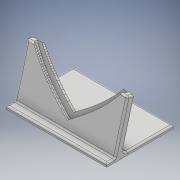
# Autodesk Inventor part: Supporto5
Saved by Autodesk Inventor 2018 (Build 220112000, 112)
## iProperties
Created: 2020-01-19
Part Number: Supporto5
Material: Generic
Document SubType Name: Modeling
Designer: Lorenzo Spadaro
Density: 1 g/cm^3
Appearance: Default
Author: Lorenzo Spadaro
Autodesk Inventor part; units mm, degrees
ref_plane "YZ Plane" through (0, 0, 0) normal (1, 0, 0) x (0, 1, 0)
ref_plane "XZ Plane" through (0, 0, 0) normal (0, 1, 0) x (-1, 0, 0)
ref_plane "XY Plane" through (0, 0, 0) normal (0, 0, 1) x (1, 0, 0)
sketch "Sketch1" plane through (0, 0, 0) normal (0, 0, 1) x (1, 0, 0)
  line L0 (-30, -20) -> (30, -20)
  line L1 (30, -20) -> (30, 20)
  line L2 (30, 20) -> (-30, 20)
  line L3 (-30, 20) -> (-30, -20)
  line L4 (-30, -20) -> (30, 20) construction
  line L5 (30, -20) -> (-30, 20) construction
  point P0 (0, 0)
  dimension "d0" = 60
  dimension "d1" = 40
  constraints: 12 end point, 2 midpoint, 2 parallel, 1 horizontal, 1 perpendicular
  measures "d0" distance of L2.end L1.end
  measures "d1" distance of L1.end L0.end
extrude "Extrusion1" add sketch "Sketch1" along normal blind 3
sketch "Sketch2" plane through (-30, -20, 0) normal (-1, 0, 0) x (0, 0, 1)
  line L0 (0, 0) -> (0, 40)
  line L1 (3, 40) -> (0, 40)
  line L2 (0, 40) -> (0, 0)
  line L3 (0, 0) -> (3, 0)
  line L4 (0, 40) -> (0, 20)
  line L5 (3, 40) -> (3, 5)
  line L6 (3, 5) -> (0, 5)
  line L7 (3, 0) -> (3, 40)
  line L8 (3, 5) -> (3, 0)
  line L9 (3, 5) -> (3, 9.805)
  line L10 (3, 9.805) -> (6, 9.805) construction
  line L11 (6.282765, 5.879614) -> (3, 5)
  line L12 (6.282765, 5.879614) -> (5.230961, 9.805)
  line L13 (6.282765, 5.879614) -> (10.346623, 5.879614) construction
  line L14 (5.230961, 9.805) -> (3, 9.805)
  dimension "d5" = 35
  dimension "d19" = 105
  dimension "d26" = 4.805
  dimension "d27" = 105
  constraints: 26 end point, 3 collinear, 3 horizontal, 3 point on line, 2 perpendicular, 1 equal length, 1 vertical
  measures "d5" distance of L1.start L5.end
  measures "d19" angle of L13 L12
  measures "d26" distance from line of L5.end L10
  measures "d27" angle of L7 L11
extrude "Extrusion2" add sketch "Sketch2" against normal blind 60 contours L5 L14 L12 L11
sketch "Sketch3" plane through (-30, -15, 3) normal (0, -0.9659258, 0.258819) x (1, 0, 0)
  line L0 (0, 3.398568) -> (60, 3.398568)
  line L1 (12.592311, 64.303412) -> (12.958694, 64.332521)
  line L2 (12.958694, 64.332521) -> (15.177373, 64.415061)
  line L3 (15.177373, 64.415061) -> (16.661991, 64.365177)
  line L4 (16.661991, 64.365177) -> (17.769726, 64.261939)
  line L5 (17.769726, 64.261939) -> (18.867022, 64.095258)
  line L6 (18.867022, 64.095258) -> (19.590244, 63.945636)
  line L7 (19.590244, 63.945636) -> (20.305002, 63.763178)
  line L8 (20.305002, 63.763178) -> (21.009903, 63.54578)
  line L9 (21.009903, 63.54578) -> (21.703356, 63.291635)
  line L10 (21.703356, 63.291635) -> (22.383868, 62.998836)
  line L11 (22.383868, 62.998836) -> (23.049947, 62.665577)
  line L12 (23.049947, 62.665577) -> (23.331467, 62.515535)
  line L13 (23.331467, 62.515535) -> (24.149779, 62.028902)
  line L14 (24.149779, 62.028902) -> (25.185077, 61.30316)
  line L15 (25.185077, 61.30316) -> (26.400848, 60.29306)
  line L16 (26.400848, 60.29306) -> (29.885544, 56.611384)
  line L17 (29.885544, 56.611384) -> (33.703552, 60.647146)
  line L18 (33.703552, 60.647146) -> (35.076276, 61.73641)
  line L19 (35.076276, 61.73641) -> (36.056629, 62.380953)
  line L20 (36.056629, 62.380953) -> (36.398998, 62.583466)
  line L21 (36.398998, 62.583466) -> (36.746215, 62.774297)
  line L22 (36.746215, 62.774297) -> (37.098078, 62.953848)
  line L23 (37.098078, 62.953848) -> (37.454288, 63.122217)
  line L24 (37.454288, 63.122217) -> (37.814542, 63.279703)
  line L25 (37.814542, 63.279703) -> (38.54658, 63.563221)
  line L26 (38.54658, 63.563221) -> (39.292386, 63.806195)
  line L27 (39.292386, 63.806195) -> (40.050049, 64.010818)
  line L28 (40.050049, 64.010818) -> (40.817863, 64.178882)
  line L29 (40.817863, 64.178882) -> (41.59382, 64.31238)
  line L30 (41.59382, 64.31238) -> (42.376111, 64.413403)
  line L31 (42.376111, 64.413403) -> (43.55743, 64.50827)
  line L32 (43.55743, 64.50827) -> (45.137415, 64.539379)
  line L33 (45.137415, 64.539379) -> (47.099711, 64.447361)
  line L34 (47.099711, 64.447361) -> (47.482254, 64.413437)
  line L35 (47.482254, 64.413437) -> (47.862944, 64.368005)
  line L36 (47.862944, 64.368005) -> (48.24148, 64.311464)
  line L37 (48.24148, 64.311464) -> (48.991688, 64.165553)
  line L38 (48.991688, 64.165553) -> (49.73137, 63.977198)
  line L39 (49.73137, 63.977198) -> (50.45922, 63.748095)
  line L40 (50.45922, 63.748095) -> (51.173731, 63.479836)
  line L41 (51.173731, 63.479836) -> (51.873497, 63.174016)
  line L42 (51.873497, 63.174016) -> (52.55711, 62.832229)
  line L43 (52.55711, 62.832229) -> (53.223066, 62.456069)
  line L44 (53.223066, 62.456069) -> (53.870055, 62.047231)
  line L45 (53.870055, 62.047231) -> (54.496573, 61.607208)
  line L46 (54.496573, 61.607208) -> (55.101212, 61.137695)
  line L47 (55.101212, 61.137695) -> (55.682567, 60.640185)
  line L48 (55.682567, 60.640185) -> (56.239229, 60.116474)
  line L49 (56.239229, 60.116474) -> (56.769693, 59.567954)
  line L50 (56.769693, 59.567954) -> (57.086721, 59.221957)
  line L51 (57.086721, 59.221957) -> (57.393082, 58.867816)
  line L52 (57.393082, 58.867816) -> (57.688776, 58.505831)
  line L53 (57.688776, 58.505831) -> (57.973892, 58.136396)
  line L54 (57.973892, 58.136396) -> (58.248465, 57.759638)
  line L55 (58.248465, 57.759638) -> (58.512767, 57.376037)
  line L56 (58.512767, 57.376037) -> (58.766597, 56.985692)
  line L57 (58.766597, 56.985692) -> (59.010253, 56.589105)
  line L58 (59.010253, 56.589105) -> (59.243835, 56.186375)
  line L59 (59.243835, 56.186375) -> (59.46724, 55.777903)
  line L60 (59.46724, 55.777903) -> (59.680669, 55.36389)
  line L61 (59.680669, 55.36389) -> (60.077988, 54.520739)
  line L62 (60.077988, 54.520739) -> (60.436185, 53.659126)
  line L63 (60.436185, 53.659126) -> (60.756147, 52.781552)
  line L64 (60.756147, 52.781552) -> (61.038466, 51.890322)
  line L65 (61.038466, 51.890322) -> (61.283833, 50.987737)
  line L66 (61.283833, 50.987737) -> (61.492836, 50.076101)
  line L67 (61.492836, 50.076101) -> (61.666167, 49.157916)
  line L68 (61.666167, 49.157916) -> (61.804515, 48.235385)
  line L69 (61.804515, 48.235385) -> (61.908472, 47.31091)
  line L70 (61.908472, 47.31091) -> (61.925428, 43.259027)
  line L71 (61.925428, 43.259027) -> (61.867686, 42.674287)
  line L72 (61.867686, 42.674287) -> (61.795735, 42.088881)
  line L73 (61.795735, 42.088881) -> (61.710172, 41.506318)
  line L74 (61.710172, 41.506318) -> (61.611397, 40.9266)
  line L75 (61.611397, 40.9266) -> (61.49971, 40.349827)
  line L76 (61.49971, 40.349827) -> (61.37541, 39.776102)
  line L77 (61.37541, 39.776102) -> (61.238797, 39.205425)
  line L78 (61.238797, 39.205425) -> (61.09027, 38.637999)
  line L79 (61.09027, 38.637999) -> (60.92993, 38.073723)
  line L80 (60.92993, 38.073723) -> (60.758376, 37.5127)
  line L81 (60.758376, 37.5127) -> (60.575708, 36.955031)
  line L82 (60.575708, 36.955031) -> (60.178429, 35.850058)
  line L83 (60.178429, 35.850058) -> (59.740789, 34.759417)
  line L84 (59.740789, 34.759417) -> (59.265187, 33.683618)
  line L85 (59.265187, 33.683618) -> (58.754121, 32.62307)
  line L86 (58.754121, 32.62307) -> (58.210087, 31.578484)
  line L87 (58.210087, 31.578484) -> (57.635685, 30.550371)
  line L88 (57.635685, 30.550371) -> (56.722496, 29.040236)
  line L89 (56.722496, 29.040236) -> (55.754839, 27.570274)
  line L90 (55.754839, 27.570274) -> (55.262169, 26.869206)
  line L91 (55.262169, 26.869206) -> (54.759665, 26.176097)
  line L92 (54.759665, 26.176097) -> (54.247729, 25.490649)
  line L93 (54.247729, 25.490649) -> (53.726461, 24.812762)
  line L94 (53.726461, 24.812762) -> (53.196262, 24.142237)
  line L95 (53.196262, 24.142237) -> (52.110275, 22.822781)
  line L96 (52.110275, 22.822781) -> (50.991771, 21.530989)
  line L97 (50.991771, 21.530989) -> (49.843056, 20.265571)
  line L98 (49.843056, 20.265571) -> (48.666436, 19.025336)
  line L99 (48.666436, 19.025336) -> (47.464115, 17.808994)
  line L100 (47.464115, 17.808994) -> (45.617358, 16.02655)
  line L101 (45.617358, 16.02655) -> (43.725406, 14.290617)
  line L102 (43.725406, 14.290617) -> (40.492299, 11.489663)
  line L103 (40.492299, 11.489663) -> (38.516713, 9.857281)
  line L104 (38.516713, 9.857281) -> (30.108542, 3.524339)
  line L105 (30.108542, 3.524339) -> (25.613236, 6.766256)
  line L106 (25.613236, 6.766256) -> (22.956408, 8.774555)
  line L107 (22.956408, 8.774555) -> (21.20846, 10.144353)
  line L108 (21.20846, 10.144353) -> (19.4827, 11.541243)
  line L109 (19.4827, 11.541243) -> (17.782216, 12.967639)
  line L110 (17.782216, 12.967639) -> (16.1101, 14.425454)
  line L111 (16.1101, 14.425454) -> (15.28559, 15.166911)
  line L112 (15.28559, 15.166911) -> (14.469444, 15.917102)
  line L113 (14.469444, 15.917102) -> (13.66186, 16.676229)
  line L114 (13.66186, 16.676229) -> (12.863337, 17.444594)
  line L115 (12.863337, 17.444594) -> (12.074175, 18.222498)
  line L116 (12.074175, 18.222498) -> (11.294772, 19.010244)
  line L117 (11.294772, 19.010244) -> (10.525626, 19.808032)
  line L118 (10.525626, 19.808032) -> (9.767038, 20.616064)
  line L119 (9.767038, 20.616064) -> (9.019406, 21.434743)
  line L120 (9.019406, 21.434743) -> (8.283128, 22.264369)
  line L121 (8.283128, 22.264369) -> (7.558503, 23.105044)
  line L122 (7.558503, 23.105044) -> (6.846031, 23.95717)
  line L123 (6.846031, 23.95717) -> (6.14611, 24.821048)
  line L124 (6.14611, 24.821048) -> (5.295269, 25.928197)
  line L125 (5.295269, 25.928197) -> (4.470723, 27.060657)
  line L126 (4.470723, 27.060657) -> (3.676074, 28.217642)
  line L127 (3.676074, 28.217642) -> (2.915326, 29.398568)
  line L128 (2.915326, 29.398568) -> (2.548714, 29.997939)
  line L129 (2.548714, 29.997939) -> (2.192079, 30.603052)
  line L130 (2.192079, 30.603052) -> (1.845719, 31.213908)
  line L131 (1.845719, 31.213908) -> (1.510336, 31.83041)
  line L132 (1.510336, 31.83041) -> (1.186131, 32.452459)
  line L133 (1.186131, 32.452459) -> (0.873701, 33.080057)
  line L134 (0.873701, 33.080057) -> (0.57365, 33.713107)
  line L135 (0.57365, 33.713107) -> (0.286176, 34.351509)
  line L136 (0.286176, 34.351509) -> (0.01208, 34.995168)
  line L137 (0.01208, 34.995168) -> (-0.248439, 35.644183)
  line L138 (-0.248439, 35.644183) -> (-0.494778, 36.298258)
  line L139 (-0.494778, 36.298258) -> (-0.726439, 36.957495)
  line L140 (-0.726439, 36.957495) -> (-0.94302, 37.621694)
  line L141 (-0.94302, 37.621694) -> (-1.144022, 38.290859)
  line L142 (-1.144022, 38.290859) -> (-1.328845, 38.964891)
  line L143 (-1.328845, 38.964891) -> (-1.497187, 39.643693)
  line L144 (-1.497187, 39.643693) -> (-1.648549, 40.327365)
  line L145 (-1.648549, 40.327365) -> (-1.78243, 41.015611)
  line L146 (-1.78243, 41.015611) -> (-1.898231, 41.708532)
  line L147 (-1.898231, 41.708532) -> (-1.99565, 42.405931)
  line L148 (-1.99565, 42.405931) -> (-2.074088, 43.107809)
  line L149 (-2.074088, 43.107809) -> (-2.089544, 46.801076)
  line L150 (-2.089544, 46.801076) -> (-1.961684, 48.029622)
  line L151 (-1.961684, 48.029622) -> (-1.776004, 49.25341)
  line L152 (-1.776004, 49.25341) -> (-1.530382, 50.467349)
  line L153 (-1.530382, 50.467349) -> (-1.222497, 51.666447)
  line L154 (-1.222497, 51.666447) -> (-0.85023, 52.846016)
  line L155 (-0.85023, 52.846016) -> (-0.565162, 53.619015)
  line L156 (-0.565162, 53.619015) -> (-0.249943, 54.379641)
  line L157 (-0.249943, 54.379641) -> (0.096236, 55.126296)
  line L158 (0.096236, 55.126296) -> (0.473978, 55.857784)
  line L159 (0.473978, 55.857784) -> (0.883891, 56.572405)
  line L160 (0.883891, 56.572405) -> (1.326681, 57.268764)
  line L161 (1.326681, 57.268764) -> (1.802953, 57.945463)
  line L162 (1.802953, 57.945463) -> (2.070477, 58.298886)
  line L163 (2.070477, 58.298886) -> (2.347528, 58.645648)
  line L164 (2.347528, 58.645648) -> (2.634008, 58.98545)
  line L165 (2.634008, 58.98545) -> (2.929719, 59.317991)
  line L166 (2.929719, 59.317991) -> (3.234362, 59.642968)
  line L167 (3.234362, 59.642968) -> (3.547638, 59.960082)
  line L168 (3.547638, 59.960082) -> (3.869349, 60.268831)
  line L169 (3.869349, 60.268831) -> (4.199195, 60.569114)
  line L170 (4.199195, 60.569114) -> (4.537079, 60.860431)
  line L171 (4.537079, 60.860431) -> (4.882701, 61.142479)
  line L172 (4.882701, 61.142479) -> (5.235764, 61.414959)
  line L173 (5.235764, 61.414959) -> (5.595969, 61.677469)
  line L174 (5.595969, 61.677469) -> (5.963333, 61.929784)
  line L175 (5.963333, 61.929784) -> (6.33734, 62.171527)
  line L176 (6.33734, 62.171527) -> (6.717792, 62.402396)
  line L177 (6.717792, 62.402396) -> (7.104591, 62.621991)
  line L178 (7.104591, 62.621991) -> (7.497437, 62.830012)
  line L179 (7.497437, 62.830012) -> (7.896033, 63.026155)
  line L180 (7.896033, 63.026155) -> (8.300079, 63.210021)
  line L181 (8.300079, 63.210021) -> (8.709476, 63.381409)
  line L182 (8.709476, 63.381409) -> (9.123927, 63.539818)
  line L183 (9.123927, 63.539818) -> (9.543232, 63.685046)
  line L184 (9.543232, 63.685046) -> (9.966994, 63.816693)
  line L185 (9.966994, 63.816693) -> (10.395212, 63.934458)
  line L186 (10.395212, 63.934458) -> (10.827389, 64.038039)
  line L187 (10.827389, 64.038039) -> (11.263526, 64.127036)
  line L188 (11.263526, 64.127036) -> (11.703125, 64.201148)
  line L189 (11.703125, 64.201148) -> (12.146186, 64.260074)
  line L190 (12.146186, 64.260074) -> (12.592311, 64.303412)
  line L191 (0, 0) -> (0, 3.398568)
  line L192 (0, 3.398568) -> (0, 29.398568)
  line L193 (0, 29.398568) -> (2.915326, 29.398568)
  line L194 (60, 3.398568) -> (60, 0)
  line L195 (60, 3.398568) -> (60, 29.398568)
  line L196 (60, 29.398568) -> (56.939182, 29.398568)
  point P0 (30, 0.984508)
  dimension "d15" = 26
  dimension "d16" = 26
  constraints: 388 end point, 4 perpendicular, 2 point on line, 1 horizontal, 1 parallel, 1 vertical
  measures "d15" distance of L0.start L192.end
  measures "d16" distance of L0.end L195.end
extrude "Extrusion3" add sketch "Sketch3" against normal blind 3.1 contours L192 L193 L127 L126 L125 L124 L123 L122 L121 L120 L119 L118 L117 L116 L115 L114 L113 L112 L111 L110 L109 L108 L107 L106 L105 L104 L103 L102 L101 L100 L99 L98 L97 L96 L95 L94 L93 L92 L91 L90 L89 L88 L196 L195 L0
sketch "Sketch4" plane through (26.939182, -7.391091, 31.396836) normal (0, 0.258819, 0.9659258) x (1, 0, 0)
  line L0 (3.060818, 3.1) -> (3.060818, 3.1)
  line L1 (-56.939182, 3.1) -> (-56.939182, 3.1)
  line L2 (-56.939182, 3.1) -> (3.060818, 3.1)
  line L3 (-56.939182, 5.40781) -> (3.060818, 5.40781)
  line L4 (-56.939182, 3.1) -> (-56.939182, 4.6)
  line L5 (-56.939182, 34.583861) -> (-56.939182, -4.053172)
  line L6 (-56.939182, 4.6) -> (3.060818, 4.6)
  line L7 (3.060818, 4.6) -> (3.060818, 3.1)
  line L8 (3.060818, -4.053172) -> (3.060818, 34.583861)
  point P0 (-26.939182, 15.265345)
  point P1 (-56.939182, 4.641274)
  point P2 (3.060818, 4.641274)
  dimension "d23" = 1.5
  constraints: 8 end point, 1 collinear, 1 perpendicular, 1 point on line
  measures "d23" distance of L1.start L4.end
extrude "Extrusion5" add sketch "Sketch4" against normal blind 28 contours L4 L6 L7 L2
sketch "Sketch6" plane through (-27.084674, -4.396721, 30.594497) normal (0, -0.9659258, 0.258819) x (1, 0, 0)
  line L0 (0, 0) -> (0.760749, -1.180927)
  line L1 (0.760749, -1.180927) -> (1.555397, -2.337911)
  line L2 (1.555397, -2.337911) -> (2.379944, -3.470371)
  line L3 (0, 0) -> (0.760749, -1.180927)
  line L4 (0.760749, -1.180927) -> (1.555397, -2.337911)
  line L5 (1.555397, -2.337911) -> (2.379944, -3.470371)
  line L6 (2.379944, -3.470371) -> (3.230784, -4.57752)
  line L7 (3.230784, -4.57752) -> (3.930705, -5.441399)
  line L8 (3.930705, -5.441399) -> (4.643178, -6.293524)
  line L9 (4.643178, -6.293524) -> (5.367802, -7.134199)
  line L10 (5.367802, -7.134199) -> (6.10408, -7.963825)
  line L11 (6.10408, -7.963825) -> (6.851713, -8.782504)
  line L12 (6.851713, -8.782504) -> (7.610301, -9.590537)
  line L13 (7.610301, -9.590537) -> (8.379446, -10.388325)
  line L14 (8.379446, -10.388325) -> (9.15885, -11.17607)
  line L15 (9.15885, -11.17607) -> (9.948012, -11.953974)
  line L16 (9.948012, -11.953974) -> (10.746534, -12.72234)
  line L17 (10.746534, -12.72234) -> (11.554118, -13.481467)
  line L18 (11.554118, -13.481467) -> (12.370265, -14.231658)
  line L19 (12.370265, -14.231658) -> (13.194775, -14.973114)
  line L20 (13.194775, -14.973114) -> (14.86689, -16.430929)
  line L21 (14.86689, -16.430929) -> (16.567374, -17.857326)
  line L22 (16.567374, -17.857326) -> (18.293135, -19.254216)
  line L23 (18.293135, -19.254216) -> (20.041082, -20.624013)
  line L24 (20.041082, -20.624013) -> (22.69791, -22.632312)
  line L25 (22.69791, -22.632312) -> (27.193216, -25.874229)
  line L26 (27.193216, -25.874229) -> (35.601388, -19.541287)
  line L27 (35.601388, -19.541287) -> (37.576974, -17.908905)
  line L28 (37.576974, -17.908905) -> (40.810081, -15.107951)
  line L29 (40.810081, -15.107951) -> (42.702033, -13.372018)
  line L30 (42.702033, -13.372018) -> (44.54879, -11.589575)
  line L31 (44.54879, -11.589575) -> (45.75111, -10.373232)
  line L32 (45.75111, -10.373232) -> (46.927731, -9.132998)
  line L33 (46.927731, -9.132998) -> (48.076445, -7.867579)
  line L34 (48.076445, -7.867579) -> (49.194949, -6.575787)
  line L35 (49.194949, -6.575787) -> (50.280937, -5.256331)
  line L36 (50.280937, -5.256331) -> (50.811136, -4.585807)
  line L37 (50.811136, -4.585807) -> (51.332403, -3.907919)
  line L38 (51.332403, -3.907919) -> (51.844339, -3.222471)
  line L39 (51.844339, -3.222471) -> (52.346843, -2.529362)
  line L40 (52.346843, -2.529362) -> (52.839514, -1.828294)
  line L41 (52.839514, -1.828294) -> (53.807171, -0.358332)
  line L42 (53.807171, -0.358332) -> (54.023856, 0)
  line L43 (0, 0) -> (54.023856, 0)
  line L44 (0, 4) -> (0.760749, 2.819073)
  line L45 (0.760749, 2.819073) -> (1.555397, 1.662089)
  line L46 (1.555397, 1.662089) -> (2.379944, 0.529629)
  line L47 (0, 4) -> (0.760749, 2.819073)
  line L48 (0.760749, 2.819073) -> (1.555397, 1.662089)
  line L49 (1.555397, 1.662089) -> (2.379944, 0.529629)
  line L50 (2.379944, 0.529629) -> (3.230784, -0.57752)
  line L51 (3.230784, -0.57752) -> (3.930705, -1.441399)
  line L52 (3.930705, -1.441399) -> (4.643178, -2.293524)
  line L53 (4.643178, -2.293524) -> (5.367802, -3.134199)
  line L54 (5.367802, -3.134199) -> (6.10408, -3.963825)
  line L55 (6.10408, -3.963825) -> (6.851713, -4.782504)
  line L56 (6.851713, -4.782504) -> (7.610301, -5.590537)
  line L57 (7.610301, -5.590537) -> (8.379446, -6.388325)
  line L58 (8.379446, -6.388325) -> (9.15885, -7.17607)
  line L59 (9.15885, -7.17607) -> (9.948012, -7.953974)
  line L60 (9.948012, -7.953974) -> (10.746534, -8.72234)
  line L61 (10.746534, -8.72234) -> (11.554118, -9.481467)
  line L62 (11.554118, -9.481467) -> (12.370265, -10.231658)
  line L63 (12.370265, -10.231658) -> (13.194775, -10.973114)
  line L64 (13.194775, -10.973114) -> (14.86689, -12.430929)
  line L65 (14.86689, -12.430929) -> (16.567374, -13.857326)
  line L66 (16.567374, -13.857326) -> (18.293135, -15.254216)
  line L67 (18.293135, -15.254216) -> (20.041082, -16.624013)
  line L68 (20.041082, -16.624013) -> (22.69791, -18.632312)
  line L69 (22.69791, -18.632312) -> (27.193216, -21.874229)
  line L70 (27.193216, -21.874229) -> (35.601388, -15.541287)
  line L71 (35.601388, -15.541287) -> (37.576974, -13.908905)
  line L72 (37.576974, -13.908905) -> (40.810081, -11.107951)
  line L73 (40.810081, -11.107951) -> (42.702033, -9.372018)
  line L74 (42.702033, -9.372018) -> (44.54879, -7.589575)
  line L75 (44.54879, -7.589575) -> (45.75111, -6.373232)
  line L76 (45.75111, -6.373232) -> (46.927731, -5.132998)
  line L77 (46.927731, -5.132998) -> (48.076445, -3.867579)
  line L78 (48.076445, -3.867579) -> (49.194949, -2.575787)
  line L79 (49.194949, -2.575787) -> (50.280937, -1.256331)
  line L80 (50.280937, -1.256331) -> (50.811136, -0.585807)
  line L81 (50.811136, -0.585807) -> (51.332403, 0.092081)
  line L82 (51.332403, 0.092081) -> (51.844339, 0.777529)
  line L83 (51.844339, 0.777529) -> (52.346843, 1.470638)
  line L84 (52.346843, 1.470638) -> (52.839514, 2.171706)
  line L85 (52.839514, 2.171706) -> (53.807171, 3.641668)
  line L86 (27.193216, -21.874229) -> (27.193216, -25.874229)
  line L87 (0, 0) -> (54.023856, 0)
  line L88 (2.786962, 0) -> (51.261597, 0)
  point P0 (27.084674, -28.41406)
  dimension "d69" = 4
  constraints: 88 end point, 4 point on line
  measures "d69" distance of L25.end L70.start
extrude "Extrusion11" cut sketch "Sketch6" against normal up to next contours L43 L81 L80 L79 L78 L77 L76 L75 L74 L73 L72 L71 L70 L69 L68 L67 L66 L65 L64 L63 L62 L61 L60 L59 L58 L57 L56 L55 L54 L53 L52 L51 L50
sketch "Sketch11" plane through (-30, -15, 3) normal (0, -0.9659258, 0.258819) x (1, 0, 0)
  line L0 (3.676074, 28.217642) -> (2.915326, 29.398568)
  line L1 (4.470723, 27.060657) -> (3.676074, 28.217642)
  line L2 (5.295269, 25.928197) -> (4.470723, 27.060657)
  line L3 (6.14611, 24.821048) -> (5.295269, 25.928197)
  line L4 (6.846031, 23.95717) -> (6.14611, 24.821048)
  line L5 (7.558503, 23.105044) -> (6.846031, 23.95717)
  line L6 (8.283128, 22.264369) -> (7.558503, 23.105044)
  line L7 (9.019406, 21.434743) -> (8.283128, 22.264369)
  line L8 (9.767038, 20.616064) -> (9.019406, 21.434743)
  line L9 (10.525626, 19.808032) -> (9.767038, 20.616064)
  line L10 (11.294772, 19.010244) -> (10.525626, 19.808032)
  line L11 (12.074175, 18.222498) -> (11.294772, 19.010244)
  line L12 (12.863337, 17.444594) -> (12.074175, 18.222498)
  line L13 (14.469444, 15.917102) -> (13.66186, 16.676229)
  line L14 (13.66186, 16.676229) -> (12.863337, 17.444594)
  line L15 (15.28559, 15.166911) -> (14.469444, 15.917102)
  line L16 (16.1101, 14.425454) -> (15.28559, 15.166911)
  line L17 (17.782216, 12.967639) -> (16.1101, 14.425454)
  line L18 (19.4827, 11.541243) -> (17.782216, 12.967639)
  line L19 (21.20846, 10.144353) -> (19.4827, 11.541243)
  line L20 (22.956408, 8.774555) -> (21.20846, 10.144353)
  line L21 (25.613236, 6.766256) -> (22.956408, 8.774555)
  line L22 (30.108542, 3.524339) -> (25.613236, 6.766256)
  line L23 (38.516713, 9.857281) -> (30.108542, 3.524339)
  line L24 (40.492299, 11.489663) -> (38.516713, 9.857281)
  line L25 (43.725406, 14.290617) -> (40.492299, 11.489663)
  line L26 (45.617358, 16.02655) -> (43.725406, 14.290617)
  line L27 (47.464115, 17.808994) -> (45.617358, 16.02655)
  line L28 (48.666436, 19.025336) -> (47.464115, 17.808994)
  line L29 (49.843056, 20.265571) -> (48.666436, 19.025336)
  line L30 (50.991771, 21.530989) -> (49.843056, 20.265571)
  line L31 (52.110275, 22.822781) -> (50.991771, 21.530989)
  line L32 (53.196262, 24.142237) -> (52.110275, 22.822781)
  line L33 (53.726461, 24.812762) -> (53.196262, 24.142237)
  line L34 (54.247729, 25.490649) -> (53.726461, 24.812762)
  line L35 (54.759665, 26.176097) -> (54.247729, 25.490649)
  line L36 (55.262169, 26.869206) -> (54.759665, 26.176097)
  line L37 (55.754839, 27.570274) -> (55.262169, 26.869206)
  line L38 (56.722496, 29.040236) -> (55.754839, 27.570274)
  line L39 (56.939182, 29.398568) -> (56.722496, 29.040236)
  line L40 (25.613236, 6.766256) -> (30.108542, 3.524339)
  line L41 (30.108542, 3.524339) -> (30.108542, 4.524339)
  line L42 (30.108542, 3.524339) -> (31.108542, 3.524339) construction
  line L43 (3.676074, 29.217642) -> (2.915326, 30.398568)
  line L44 (4.470723, 28.060657) -> (3.676074, 29.217642)
  line L45 (5.295269, 26.928197) -> (4.470723, 28.060657)
  line L46 (6.14611, 25.821048) -> (5.295269, 26.928197)
  line L47 (6.846031, 24.95717) -> (6.14611, 25.821048)
  line L48 (7.558503, 24.105044) -> (6.846031, 24.95717)
  line L49 (8.283128, 23.264369) -> (7.558503, 24.105044)
  line L50 (9.019406, 22.434743) -> (8.283128, 23.264369)
  line L51 (9.767038, 21.616064) -> (9.019406, 22.434743)
  line L52 (10.525626, 20.808032) -> (9.767038, 21.616064)
  line L53 (11.294772, 20.010244) -> (10.525626, 20.808032)
  line L54 (12.074175, 19.222498) -> (11.294772, 20.010244)
  line L55 (12.863337, 18.444594) -> (12.074175, 19.222498)
  line L56 (14.469444, 16.917102) -> (13.66186, 17.676229)
  line L57 (13.66186, 17.676229) -> (12.863337, 18.444594)
  line L58 (15.28559, 16.166911) -> (14.469444, 16.917102)
  line L59 (16.1101, 15.425454) -> (15.28559, 16.166911)
  line L60 (17.782216, 13.967639) -> (16.1101, 15.425454)
  line L61 (19.4827, 12.541243) -> (17.782216, 13.967639)
  line L62 (21.20846, 11.144353) -> (19.4827, 12.541243)
  line L63 (22.956408, 9.774555) -> (21.20846, 11.144353)
  line L64 (25.613236, 7.766256) -> (22.956408, 9.774555)
  line L65 (30.108542, 4.524339) -> (25.613236, 7.766256)
  line L66 (38.516713, 10.857281) -> (30.108542, 4.524339)
  line L67 (40.492299, 12.489663) -> (38.516713, 10.857281)
  line L68 (43.725406, 15.290617) -> (40.492299, 12.489663)
  line L69 (45.617358, 17.02655) -> (43.725406, 15.290617)
  line L70 (47.464115, 18.808994) -> (45.617358, 17.02655)
  line L71 (48.666436, 20.025336) -> (47.464115, 18.808994)
  line L72 (49.843056, 21.265571) -> (48.666436, 20.025336)
  line L73 (50.991771, 22.530989) -> (49.843056, 21.265571)
  line L74 (52.110275, 23.822781) -> (50.991771, 22.530989)
  line L75 (53.196262, 25.142237) -> (52.110275, 23.822781)
  line L76 (53.726461, 25.812762) -> (53.196262, 25.142237)
  line L77 (54.247729, 26.490649) -> (53.726461, 25.812762)
  line L78 (54.759665, 27.176097) -> (54.247729, 26.490649)
  line L79 (55.262169, 27.869206) -> (54.759665, 27.176097)
  line L80 (55.754839, 28.570274) -> (55.262169, 27.869206)
  line L81 (56.722496, 30.040236) -> (55.754839, 28.570274)
  line L82 (56.939182, 30.398568) -> (56.722496, 30.040236)
  line L83 (2.915326, 29.398568) -> (3.559522, 29.398568)
  line L84 (56.939182, 29.398568) -> (56.300094, 29.398568)
  point P0 (30, 0.984508)
  dimension "d72" = 1
  dimension "d73" = 90
  constraints: 88 end point, 3 point on line, 2 horizontal, 1 perpendicular, 1 vertical
  measures "d72" distance of L22.start L41.end
  measures "d73" angle of L42 L41
extrude "Extrusion12" add sketch "Sketch11" against normal blind 1
sketch "Sketch8" plane through (0, 0, 3) normal (0, 0, 1) x (1, 0, 0)
  line L0 (24, -5.148917) -> (21, -5.148917)
  line L1 (21, -5.148917) -> (21, -7.148917)
  line L2 (21, -7.148917) -> (24, -7.148917)
  line L3 (24, -7.148917) -> (24, -5.148917)
  line L4 (-21, -5.148917) -> (-24, -5.148917)
  line L5 (-24, -5.148917) -> (-24, -7.147451)
  line L6 (-24, -7.147451) -> (-21, -7.147451)
  line L7 (-21, -7.147451) -> (-21, -5.148917)
  line L8 (-24, -5.148917) -> (-29, -5.148917)
  line L9 (29, -5.148917) -> (24, -5.148917)
  line L10 (29, -4.877374) -> (29, 20)
  line L11 (30, 20) -> (-30, 20)
  line L12 (-29, -5.148917) -> (-29, 20)
  line L13 (30, -10.195) -> (30, 20)
  line L14 (29, -4.877374) -> (29, -5.148917)
  line L15 (29, -5.148917) -> (29, -9.566685)
  line L16 (-29, -5.148917) -> (-29, -9.566685)
  line L17 (-29, -9.566685) -> (29, -9.566685)
  line L18 (29, -9.566685) -> (30, -9.566685)
  line L19 (-29, -9.566685) -> (-30, -9.566685)
  line L20 (-30, 20) -> (-30, -10.195)
  line L21 (-29, -9.566685) -> (-28, -9.566685) construction
  point P0 (0, 0)
  dimension "d51" = 3
  dimension "d52" = 2
  dimension "d53" = 3
  dimension "d54" = 42
  dimension "d55" = 3
  dimension "d56" = 5
  dimension "d62" = 27.14745
  dimension "d63" = 24.87737
  dimension "d76" = 180
  constraints: 38 end point, 9 perpendicular, 5 point on line, 3 vertical, 2 horizontal, 1 collinear, 1 parallel
  measures "d51" distance of L0.start L0.end
  measures "d52" distance of L0.end L1.end
  measures "d53" distance of L1.end L2.end
  measures "d54" distance of L0.end L4.start
  measures "d55" distance of L4.start L4.end
  measures "d56" distance of L4.end L8.end
  measures "d62" distance between parallel lines of L6 L11
  measures "d63" distance from line of L10.start L11
  measures "d76" angle of L19 L21
extrude "Extrusion9" add sketch "Sketch8" along normal up to next contours L3 L2 L1 L0 | L7 L6 L5 L4
sketch "Sketch10" plane through (0, 0, 0) normal (0, 0, -1) x (-1, 0, 0)
  line L0 (-30, 20) -> (30, 20)
  line L1 (-30, 20) -> (-30, -20)
  line L2 (-30, -20) -> (30, -20)
  line L3 (30, 20) -> (30, -20) projected
  line L4 (30, -20) -> (30, 20)
  point P0 (0, 0)
  constraints: 8 end point, 2 perpendicular, 1 vertical
extrude "Extrusion10" cut sketch "Sketch10" against normal blind 1
fillet "Fillet7" radius 0.5 16 edges at (-21, -5.1489, 12.4959) (-21, -7.1475, 8.7665) (-24, -5.1489, 12.4959) (-24, -7.1475, 8.7665) (21, -5.1489, 12.4959) (21, -7.1489, 8.7638) (24, -5.1489, 12.4959) (24, -7.1489, 8.7638) (24, -6.1489, 3) (22.5, -7.1489, 3) (21, -6.1489, 3) (22.5, -5.1489, 3) (-24, -6.1482, 3) (-22.5, -5.1489, 3) (-21, -6.1482, 3) (-22.5, -7.1475, 3)
fillet "Fillet9" radius 2 5 edges at (0, -10.195, 3) (0, -10.1948, 3.1603) (30, -10.1949, 3.1604) (-30, -10.1949, 3.1604) (0, -10.195, 3.1604)
fillet "Fillet10" radius 1 18 edges at (-30, 6.1844, 3) (-30, -6.2555, 17.862) (-30, -9.218, 3.7825) (0, 20, 3) (-30, -11.1955, 17.1984) (-30, -17.5, 3) (30, -9.218, 3.7825) (30, -6.2555, 17.862) (30, 6.1844, 3) (30, -17.5, 3) (0, -20, 3) (-28.2202, -7.3911, 31.3968) (-27.1489, -2.9478, 30.2063) (28.15, -7.3911, 31.3968) (30, -5.1695, 30.8016) (27.0885, -2.9478, 30.2063) (0, -15, 3) (30, -11.1955, 17.1984)
body "Solid1"
